Autodesk Inventor part; units mm, degrees
(part 3 of 3)
  line L418 (-54.6413, 55.359) -> (-49.6413, 64.0192) projected
  line L419 (-64.6413, 55.359) -> (-54.6413, 55.359) projected
  line L420 (-69.6413, 64.0192) -> (-64.6413, 55.359) projected
  line L421 (-64.6413, 72.6795) -> (-69.6413, 64.0192) projected
  line L422 (-25.981, 77.6795) -> (-15.981, 77.6795) projected
  line L423 (-30.981, 86.3397) -> (-25.981, 77.6795) projected
  line L424 (-25.981, 95) -> (-30.981, 86.3397) projected
  line L425 (-15.981, 95) -> (-25.981, 95) projected
  line L426 (-10.981, 86.3397) -> (-15.981, 95) projected
  line L427 (-15.981, 77.6795) -> (-10.981, 86.3397) projected
  line L428 (66.3397, 64.0192) -> (61.3397, 72.6795) projected
  line L429 (61.3397, 55.359) -> (66.3397, 64.0192) projected
  line L430 (51.3397, 55.359) -> (61.3397, 55.359) projected
  line L431 (46.3397, 64.0192) -> (51.3397, 55.359) projected
  line L432 (51.3397, 72.6795) -> (46.3397, 64.0192) projected
  line L433 (61.3397, 72.6795) -> (51.3397, 72.6795) projected
  line L434 (90, 77.6795) -> (100, 77.6795) projected
  line L435 (85, 86.3397) -> (90, 77.6795) projected
  line L436 (90, 95) -> (85, 86.3397) projected
  line L437 (100, 95) -> (90, 95) projected
  line L438 (105, 86.3397) -> (100, 95) projected
  line L439 (100, 77.6795) -> (105, 86.3397) projected
  line L440 (22.6795, 33.0382) -> (27.6795, 41.6985) projected
  line L441 (12.6795, 33.0382) -> (22.6795, 33.0382) projected
  line L442 (7.6795, 41.6985) -> (12.6795, 33.0382) projected
  line L443 (12.6795, 50.3587) -> (7.6795, 41.6985) projected
  line L444 (22.6795, 50.3587) -> (12.6795, 50.3587) projected
  line L445 (27.6795, 41.6985) -> (22.6795, 50.3587) projected
  line L446 (61.3399, 33.0382) -> (66.3399, 41.6985) projected
  line L447 (51.3399, 33.0382) -> (61.3399, 33.0382) projected
  line L448 (46.3399, 41.6985) -> (51.3399, 33.0382) projected
  line L449 (51.3399, 50.3587) -> (46.3399, 41.6985) projected
  line L450 (61.3399, 50.3587) -> (51.3399, 50.3587) projected
  line L451 (66.3399, 41.6985) -> (61.3399, 50.3587) projected
  line L452 (-11.6509, 75.1795) -> (-6.6509, 66.5192) projected
  line L453 (-6.6509, 83.8397) -> (-11.6509, 75.1795) projected
  line L454 (3.3491, 83.8397) -> (-6.6509, 83.8397) projected
  line L455 (8.3491, 75.1795) -> (3.3491, 83.8397) projected
  line L456 (3.3491, 66.5192) -> (8.3491, 75.1795) projected
  line L457 (-6.6509, 66.5192) -> (3.3491, 66.5192) projected
  line L458 (-45.3111, 83.8397) -> (-50.3111, 75.1795) projected
  line L459 (-35.3111, 83.8397) -> (-45.3111, 83.8397) projected
  line L460 (-30.3111, 75.1795) -> (-35.3111, 83.8397) projected
  line L461 (-35.3111, 66.5192) -> (-30.3111, 75.1795) projected
  line L462 (-45.3111, 66.5192) -> (-35.3111, 66.5192) projected
  line L463 (-50.3111, 75.1795) -> (-45.3111, 66.5192) projected
  line L464 (42.0096, 66.5192) -> (47.0096, 75.1795) projected
  line L465 (32.0096, 66.5192) -> (42.0096, 66.5192) projected
  line L466 (27.0096, 75.1795) -> (32.0096, 66.5192) projected
  line L467 (32.0096, 83.8397) -> (27.0096, 75.1795) projected
  line L468 (42.0096, 83.8397) -> (32.0096, 83.8397) projected
  line L469 (47.0096, 75.1795) -> (42.0096, 83.8397) projected
  line L470 (80.6699, 66.5192) -> (85.6699, 75.1795) projected
  line L471 (70.6699, 66.5192) -> (80.6699, 66.5192) projected
  line L472 (65.6699, 75.1795) -> (70.6699, 66.5192) projected
  line L473 (70.6699, 83.8397) -> (65.6699, 75.1795) projected
  line L474 (80.6699, 83.8397) -> (70.6699, 83.8397) projected
  line L475 (85.6699, 75.1795) -> (80.6699, 83.8397) projected
  line L476 (22.6795, 72.6795) -> (12.6795, 72.6795) projected
  line L477 (27.6795, 64.0192) -> (22.6795, 72.6795) projected
  line L478 (22.6795, 55.359) -> (27.6795, 64.0192) projected
  line L479 (12.6795, 55.359) -> (22.6795, 55.359) projected
  line L480 (7.6795, 64.0192) -> (12.6795, 55.359) projected
  line L481 (12.6795, 72.6795) -> (7.6795, 64.0192) projected
  line L482 (-22.75, -78.5665) -> (-17.25, -78.5665) projected
  line L483 (-22.75, -78.566) -> (-22.75, -78.5665) projected
  line L484 (-25.981, -78.566) -> (-22.75, -78.566) projected
  line L485 (-30.981, -69.9058) -> (-25.981, -78.566) projected
  line L486 (-25.981, -61.2455) -> (-30.981, -69.9058) projected
  line L487 (-15.981, -61.2455) -> (-25.981, -61.2455) projected
  line L488 (-10.981, -69.9058) -> (-15.981, -61.2455) projected
  line L489 (-15.981, -78.566) -> (-10.981, -69.9058) projected
  line L490 (-17.25, -78.566) -> (-15.981, -78.566) projected
  line L491 (-64.6413, -78.566) -> (-54.6413, -78.566) projected
  line L492 (-69.6413, -69.9058) -> (-64.6413, -78.566) projected
  line L493 (-64.6413, -61.2455) -> (-69.6413, -69.9058) projected
  line L494 (-54.6413, -61.2455) -> (-64.6413, -61.2455) projected
  line L495 (-49.6413, -69.9058) -> (-54.6413, -61.2455) projected
  line L496 (-54.6413, -78.566) -> (-49.6413, -69.9058) projected
  line L497 (-103.3015, -78.566) -> (-93.3015, -78.566) projected
  line L498 (-108.3015, -69.9058) -> (-103.3015, -78.566) projected
  line L499 (-103.3015, -61.2455) -> (-108.3015, -69.9058) projected
  line L500 (-93.3015, -61.2455) -> (-103.3015, -61.2455) projected
  line L501 (-88.3015, -69.9058) -> (-93.3015, -61.2455) projected
  line L502 (-93.3015, -78.566) -> (-88.3015, -69.9058) projected
  line L503 (-93.3015, -83.5665) -> (-103.3015, -83.5665) projected
  line L504 (-88.3015, -92.2268) -> (-93.3015, -83.5665) projected
  line L505 (-92.7894, -100) -> (-88.3015, -92.2268) projected
  line L506 (-65.1534, -100) -> (-92.7894, -100) projected
  line L507 (-83.9714, -94.7273) -> (-87.0156, -100) projected
  line L508 (-73.9714, -94.7273) -> (-83.9714, -94.7273) projected
  line L509 (-70.9272, -100) -> (-73.9714, -94.7273) projected
  line L510 (-65.1534, -100) -> (-92.7894, -100) projected
  line L511 (-69.6413, -92.2268) -> (-65.1534, -100) projected
  line L512 (-64.6413, -83.5665) -> (-69.6413, -92.2268) projected
  line L513 (-54.6413, -83.5665) -> (-64.6413, -83.5665) projected
  line L514 (-49.6413, -92.2268) -> (-54.6413, -83.5665) projected
  line L515 (-54.1291, -100) -> (-49.6413, -92.2268) projected
  line L516 (-65.1534, -100) -> (-54.1291, -100) projected
  line L517 (-45.3111, -94.7273) -> (-48.3553, -100) projected
  line L518 (-35.3111, -94.7273) -> (-45.3111, -94.7273) projected
  line L519 (-32.2669, -100) -> (-35.3111, -94.7273) projected
  line L520 (-26.4931, -100) -> (-92.7894, -100) projected
  line L521 (-30.981, -92.2268) -> (-26.4931, -100) projected
  line L522 (-25.981, -83.5665) -> (-30.981, -92.2268) projected
  line L523 (-15.981, -83.5665) -> (-25.981, -83.5665) projected
  line L524 (-10.981, -92.2268) -> (-15.981, -83.5665) projected
  line L525 (-15.4689, -100) -> (-10.981, -92.2268) projected
  line L526 (-65.1534, -100) -> (-15.4689, -100) projected
  line L527 (-6.6509, -94.7273) -> (-9.6951, -100) projected
  line L528 (3.3491, -94.7273) -> (-6.6509, -94.7273) projected
  line L529 (6.3933, -100) -> (3.3491, -94.7273) projected
  line L530 (12.1674, -100) -> (-92.7894, -100) projected
  line L531 (7.6795, -92.2268) -> (12.1674, -100) projected
  line L532 (12.6795, -83.5665) -> (7.6795, -92.2268) projected
  line L533 (22.6795, -83.5665) -> (12.6795, -83.5665) projected
  line L534 (27.6795, -92.2268) -> (22.6795, -83.5665) projected
  line L535 (23.1916, -100) -> (27.6795, -92.2268) projected
  line L536 (-65.1534, -100) -> (23.1916, -100) projected
  line L537 (32.0096, -94.7273) -> (28.9654, -100) projected
  line L538 (42.0096, -94.7273) -> (32.0096, -94.7273) projected
  line L539 (45.0538, -100) -> (42.0096, -94.7273) projected
  line L540 (50.8276, -100) -> (-92.7894, -100) projected
  line L541 (46.3397, -92.2268) -> (50.8276, -100) projected
  line L542 (51.3397, -83.5665) -> (46.3397, -92.2268) projected
  line L543 (61.3397, -83.5665) -> (51.3397, -83.5665) projected
  line L544 (66.3397, -92.2268) -> (61.3397, -83.5665) projected
  line L545 (61.8519, -100) -> (66.3397, -92.2268) projected
  line L546 (-65.1534, -100) -> (61.8519, -100) projected
  line L547 (70.6699, -94.7273) -> (67.6257, -100) projected
  line L548 (80.6699, -94.7273) -> (70.6699, -94.7273) projected
  line L549 (83.7141, -100) -> (80.6699, -94.7273) projected
  line L550 (89.4879, -100) -> (-92.7894, -100) projected
  line L551 (85, -92.2268) -> (89.4879, -100) projected
  line L552 (90, -83.5665) -> (85, -92.2268) projected
  line L553 (100, -83.5665) -> (90, -83.5665) projected
  line L554 (105, -92.2268) -> (100, -83.5665) projected
  line L555 (100.5121, -100) -> (105, -92.2268) projected
  line L556 (-65.1534, -100) -> (100.5121, -100) projected
  line L557 (109.3301, -94.7273) -> (106.2859, -100) projected
  line L558 (110, -94.7273) -> (109.3301, -94.7273) projected
  line L559 (110, 100) -> (110, -100) projected
  line L560 (109.3301, -89.7268) -> (110, -89.7268) projected
  line L561 (104.3301, -81.0665) -> (109.3301, -89.7268) projected
  line L562 (109.3301, -72.4063) -> (104.3301, -81.0665) projected
  line L563 (110, -72.4063) -> (109.3301, -72.4063) projected
  line L564 (110, 100) -> (110, -100) projected
  line L565 (109.3301, -67.4058) -> (110, -67.4058) projected
  line L566 (104.3301, -58.7455) -> (109.3301, -67.4058) projected
  line L567 (109.3301, -50.0853) -> (104.3301, -58.7455) projected
  line L568 (110, -50.0853) -> (109.3301, -50.0853) projected
  line L569 (110, 100) -> (110, -100) projected
  line L570 (109.3301, -45.0848) -> (110, -45.0848) projected
  line L571 (104.3301, -36.4245) -> (109.3301, -45.0848) projected
  line L572 (109.3301, -27.7643) -> (104.3301, -36.4245) projected
  line L573 (110, -27.7643) -> (109.3301, -27.7643) projected
  line L574 (110, 100) -> (110, -100) projected
  line L575 (109.3301, -22.7638) -> (110, -22.7638) projected
  line L576 (104.3301, -14.1035) -> (109.3301, -22.7638) projected
  line L577 (109.3301, -5.4433) -> (104.3301, -14.1035) projected
  line L578 (110, -5.4433) -> (109.3301, -5.4433) projected
  line L579 (110, 100) -> (110, -100) projected
  line L580 (109.3301, -0.4428) -> (110, -0.4428) projected
  line L581 (104.3301, 8.2175) -> (109.3301, -0.4428) projected
  line L582 (109.3301, 16.8777) -> (104.3301, 8.2175) projected
  line L583 (110, 16.8777) -> (109.3301, 16.8777) projected
  line L584 (110, 100) -> (110, -100) projected
  line L585 (109.3301, 21.8777) -> (110, 21.8777) projected
  line L586 (104.3301, 30.538) -> (109.3301, 21.8777) projected
  line L587 (109.3301, 39.1983) -> (104.3301, 30.538) projected
  line L588 (110, 39.1983) -> (109.3301, 39.1983) projected
  line L589 (110, 100) -> (110, -100) projected
  line L590 (109.3301, 44.1987) -> (110, 44.1987) projected
  line L591 (104.3301, 52.859) -> (109.3301, 44.1987) projected
  line L592 (109.3301, 61.5192) -> (104.3301, 52.859) projected
  line L593 (110, 61.5192) -> (109.3301, 61.5192) projected
  line L594 (110, 100) -> (110, -100) projected
  line L595 (109.3301, 66.5192) -> (110, 66.5192) projected
  line L596 (104.3301, 75.1795) -> (109.3301, 66.5192) projected
  line L597 (109.3301, 83.8397) -> (104.3301, 75.1795) projected
  line L598 (110, 83.8397) -> (109.3301, 83.8397) projected
  line L599 (110, 100) -> (110, -100) projected
  line L600 (109.3301, 88.8397) -> (110, 88.8397) projected
  line L601 (104.3301, 97.5) -> (109.3301, 88.8397) projected
  line L602 (105.7735, 100) -> (104.3301, 97.5) projected
  line L603 (84.2265, 100) -> (110, 100) projected
  line L604 (85.6699, 97.5) -> (84.2265, 100) projected
  line L605 (80.6699, 88.8397) -> (85.6699, 97.5) projected
  line L606 (70.6699, 88.8397) -> (80.6699, 88.8397) projected
  line L607 (65.6699, 97.5) -> (70.6699, 88.8397) projected
  line L608 (67.1132, 100) -> (65.6699, 97.5) projected
  line L609 (45.5662, 100) -> (67.1132, 100) projected
  line L610 (47.0096, 97.5) -> (45.5662, 100) projected
  line L611 (42.0096, 88.8397) -> (47.0096, 97.5) projected
  line L612 (32.0096, 88.8397) -> (42.0096, 88.8397) projected
  line L613 (27.0096, 97.5) -> (32.0096, 88.8397) projected
  line L614 (28.453, 100) -> (27.0096, 97.5) projected
  line L615 (6.9058, 100) -> (28.453, 100) projected
  line L616 (8.3491, 97.5) -> (6.9058, 100) projected
  line L617 (3.3491, 88.8397) -> (8.3491, 97.5) projected
  line L618 (-6.6509, 88.8397) -> (3.3491, 88.8397) projected
  line L619 (-11.6509, 97.5) -> (-6.6509, 88.8397) projected
  line L620 (-10.2075, 100) -> (-11.6509, 97.5) projected
  line L621 (-31.7545, 100) -> (-10.2075, 100) projected
  line L622 (-30.3111, 97.5) -> (-31.7545, 100) projected
  line L623 (-35.3111, 88.8397) -> (-30.3111, 97.5) projected
  line L624 (-45.3111, 88.8397) -> (-35.3111, 88.8397) projected
  line L625 (-50.3111, 97.5) -> (-45.3111, 88.8397) projected
  line L626 (-48.8678, 100) -> (-50.3111, 97.5) projected
  line L627 (-70, 100) -> (-48.8678, 100) projected
  line L628 (-70, 99.2816) -> (-70, 100) projected
  line L629 (-68.9714, 97.5) -> (-70, 99.2816) projected
  line L630 (-73.9714, 88.8397) -> (-68.9714, 97.5) projected
  line L631 (-83.9714, 88.8397) -> (-73.9714, 88.8397) projected
  line L632 (-88.9714, 97.5) -> (-83.9714, 88.8397) projected
  line L633 (-87.528, 100) -> (-88.9714, 97.5) projected
  line L634 (-93.3013, 100) -> (-87.528, 100) projected
  line L635 (-93.3014, 99.9998) -> (-93.3013, 100) projected
  line L636 (-103.3014, 99.9998) -> (-93.3014, 99.9998) projected
  line L637 (-103.3015, 100) -> (-103.3014, 99.9998) projected
  line L638 (-110, 100) -> (-103.3015, 100) projected
  line L639 (-110, 79.2821) -> (-110, 100) projected
  line L640 (-107.6314, 75.1795) -> (-110, 79.2821) projected
  line L641 (-110, 71.0769) -> (-107.6314, 75.1795) projected
  line L642 (-110, 12.3201) -> (-110, 71.0769) projected
  line L643 (-107.6314, 8.2175) -> (-110, 12.3201) projected
  line L644 (-110, 4.1149) -> (-107.6314, 8.2175) projected
  line L645 (-110, -10.0009) -> (-110, 4.1149) projected
  line L646 (-107.6314, -14.1035) -> (-110, -10.0009) projected
  line L647 (-110, -18.2061) -> (-107.6314, -14.1035) projected
  line L648 (-110, -32.3219) -> (-110, -18.2061) projected
  line L649 (-107.6314, -36.4245) -> (-110, -32.3219) projected
  line L650 (-110, -40.5271) -> (-107.6314, -36.4245) projected
  line L651 (-110, -54.6429) -> (-110, -40.5271) projected
  line L652 (-107.6314, -58.7455) -> (-110, -54.6429) projected
  line L653 (-110, -62.8481) -> (-107.6314, -58.7455) projected
  line L654 (-110, -76.9639) -> (-110, -62.8481) projected
  line L655 (-107.6314, -81.0665) -> (-110, -76.9639) projected
  line L656 (-110, -85.1691) -> (-107.6314, -81.0665) projected
  line L657 (-110, -99.2849) -> (-110, -85.1691) projected
  line L658 (-109.5872, -100) -> (-110, -99.2849) projected
  line L659 (-103.8136, -100) -> (-109.5872, -100) projected
  line L660 (-108.3015, -92.2268) -> (-103.8136, -100) projected
  line L661 (-103.3015, -83.5665) -> (-108.3015, -92.2268) projected
  line L662 (100, 72.6795) -> (90, 72.6795) projected
  line L663 (105, 64.0192) -> (100, 72.6795) projected
  line L664 (100, 55.359) -> (105, 64.0192) projected
  line L665 (90, 55.359) -> (100, 55.359) projected
  line L666 (85, 64.0192) -> (90, 55.359) projected
  line L667 (90, 72.6795) -> (85, 64.0192) projected
  line L668 (61.3397, 77.6795) -> (66.3397, 86.3397) projected
  line L669 (51.3397, 77.6795) -> (61.3397, 77.6795) projected
  line L670 (46.3397, 86.3397) -> (51.3397, 77.6795) projected
  line L671 (51.3397, 95) -> (46.3397, 86.3397) projected
  line L672 (61.3397, 95) -> (51.3397, 95) projected
  line L673 (66.3397, 86.3397) -> (61.3397, 95) projected
  line L674 (22.6795, 77.6795) -> (27.6795, 86.3397) projected
  line L675 (12.6795, 77.6795) -> (22.6795, 77.6795) projected
  line L676 (7.6795, 86.3397) -> (12.6795, 77.6795) projected
  line L677 (12.6795, 95) -> (7.6795, 86.3397) projected
  line L678 (22.6795, 95) -> (12.6795, 95) projected
  line L679 (27.6795, 86.3397) -> (22.6795, 95) projected
  line L680 (-15.981, 72.6795) -> (-25.981, 72.6795) projected
  line L681 (-10.981, 64.0192) -> (-15.981, 72.6795) projected
  line L682 (-15.981, 55.359) -> (-10.981, 64.0192) projected
  line L683 (-25.981, 55.359) -> (-15.981, 55.359) projected
  line L684 (-30.981, 64.0192) -> (-25.981, 55.359) projected
  line L685 (-25.981, 72.6795) -> (-30.981, 64.0192) projected
  line L686 (-64.6413, 77.6795) -> (-54.6413, 77.6795) projected
  line L687 (-69.6413, 86.3397) -> (-64.6413, 77.6795) projected
  line L688 (-64.6413, 95) -> (-69.6413, 86.3397) projected
  line L689 (-54.6413, 95) -> (-64.6413, 95) projected
  line L690 (-49.6413, 86.3397) -> (-54.6413, 95) projected
  line L691 (-54.6413, 77.6795) -> (-49.6413, 86.3397) projected
  line L692 (-93.3015, 72.6795) -> (-103.3015, 72.6795) projected
  line L693 (-88.3015, 64.0192) -> (-93.3015, 72.6795) projected
  line L694 (-93.3015, 55.359) -> (-88.3015, 64.0192) projected
  line L695 (-103.3015, 55.359) -> (-93.3015, 55.359) projected
  line L696 (-108.3015, 64.0192) -> (-103.3015, 55.359) projected
  line L697 (-103.3015, 72.6795) -> (-108.3015, 64.0192) projected
  line L698 (-73.9714, 39.1983) -> (-83.9714, 39.1983) projected
  line L699 (-70.4148, 33.038) -> (-73.9714, 39.1983) projected
  line L700 (-70, 33.038) -> (-70.4148, 33.038) projected
  line L701 (-70, 32.3196) -> (-70, 33.038) projected
  line L702 (-68.9714, 30.538) -> (-70, 32.3196) projected
  line L703 (-73.9714, 21.8777) -> (-68.9714, 30.538) projected
  line L704 (-83.9714, 21.8777) -> (-73.9714, 21.8777) projected
  line L705 (-88.9714, 30.538) -> (-83.9714, 21.8777) projected
  line L706 (-83.9714, 39.1983) -> (-88.9714, 30.538) projected
  line L707 (-35.3111, 39.1983) -> (-45.3111, 39.1983) projected
  line L708 (-30.3111, 30.538) -> (-35.3111, 39.1983) projected
  line L709 (-35.3111, 21.8777) -> (-30.3111, 30.538) projected
  line L710 (-45.3111, 21.8777) -> (-35.3111, 21.8777) projected
  line L711 (-50.3111, 30.538) -> (-45.3111, 21.8777) projected
  line L712 (-45.3111, 39.1983) -> (-50.3111, 30.538) projected
  line L713 (-6.6509, 44.1987) -> (3.3491, 44.1987) projected
  line L714 (-11.6509, 52.859) -> (-6.6509, 44.1987) projected
  line L715 (-6.6509, 61.5192) -> (-11.6509, 52.859) projected
  line L716 (3.3491, 61.5192) -> (-6.6509, 61.5192) projected
  line L717 (8.3491, 52.859) -> (3.3491, 61.5192) projected
  line L718 (3.3491, 44.1987) -> (8.3491, 52.859) projected
  line L719 (42.0096, 39.1983) -> (32.0096, 39.1983) projected
  line L720 (47.0096, 30.538) -> (42.0096, 39.1983) projected
  line L721 (42.0096, 21.8777) -> (47.0096, 30.538) projected
  line L722 (32.0096, 21.8777) -> (42.0096, 21.8777) projected
  line L723 (27.0096, 30.538) -> (32.0096, 21.8777) projected
  line L724 (32.0096, 39.1983) -> (27.0096, 30.538) projected
  line L725 (80.6699, 39.1983) -> (70.6699, 39.1983) projected
  line L726 (85.6699, 30.538) -> (80.6699, 39.1983) projected
  line L727 (80.6699, 21.8777) -> (85.6699, 30.538) projected
  line L728 (70.6699, 21.8777) -> (80.6699, 21.8777) projected
  line L729 (65.6699, 30.538) -> (70.6699, 21.8777) projected
  line L730 (70.6699, 39.1983) -> (65.6699, 30.538) projected
  point P0 (-70, -100)
  point P1 (-17.25, -84)
  point P2 (-17.25, -74)
  point P3 (-2.75, -39.5)
  point P4 (57.25, -79)
  point P5 (42.75, -34.5)
  point P6 (-17.25, -83.5665)
  dimension "d79" = 5
  dimension "d80" = 4.75
  dimension "d81" = 4.75
  dimension "d82" = 5
  dimension "d83" = 4.75
  dimension "d84" = 4.75
  dimension "d85" = 5
  constraints: 24 end point, 6 point on line, 5 parallel, 5 perpendicular, 4 horizontal, 3 vertical, 2 midpoint, 8 other
  measures "d79" distance between parallel lines of L2 L6
  measures "d80" distance between parallel lines of L10 L11
  measures "d81" distance from line of L12 point (-2.75, -39.5)
  measures "d82" distance between parallel lines of L12 L10
  measures "d83" distance from line of point (57.25, -79) L15
  measures "d84" distance between parallel lines of L17 L14
  measures "d85" distance between parallel lines of L15 L14
ref_plane "작업 평면1" through (0, 0, -5.5) normal (0, 0, -1) x (-1, 0, 0)
sketch "스케치5" plane through (0, 0, -5.5) normal (0, 0, -1) x (-1, 0, 0)
  line L0 (110, -95) -> (110, 95) projected
  line L1 (-70, 95) -> (-70, -95) projected
  line L2 (-7.5, -92.75) -> (-7.5, 92.75) projected
  line L3 (-70, -90.75) -> (110, -90.75)
  line L4 (110, -90.75) -> (110, -59.25)
  line L5 (110, -59.25) -> (-70, -59.25)
  line L6 (-70, -59.25) -> (-70, -90.75)
  line L7 (-70, -90.75) -> (110, -59.25) construction
  line L8 (110, -90.75) -> (-70, -59.25) construction
  arc A0 (16.25, -84) -> (23.75, -84) centre (20, -84) ccw projected
  arc A1 (23.75, -74) -> (16.25, -74) centre (20, -74) ccw projected
  circle A2 centre (-10, -69.25) radius 1.95
  circle A3 centre (-65, -64.25) radius 1.95
  circle A4 centre (-65, -95) radius 1.95
  circle A5 centre (-10, -90) radius 1.95
  line L9 (20, -111.2481) -> (20, -60.3206)
  circle A6 centre (50, -69.25) radius 1.95
  circle A7 centre (105, -64.25) radius 1.95
  circle A8 centre (105, -95) radius 1.95
  circle A9 centre (50, -90) radius 1.95
  line L10 (-65, -100) -> (105, -100) projected
  arc A10 (-63.75, -84) -> (-56.25, -84) centre (-60, -84) ccw projected
  arc A11 (-62.75, -84) -> (-57.25, -84) centre (-60, -84) ccw projected
  circle A12 centre (-10, -69.25) radius 3.5
  circle A13 centre (-10, -90) radius 3.5
  circle A14 centre (50, -69.25) radius 3.5
  circle A15 centre (50, -90) radius 3.5
  arc A16 (-70, -95) -> (-65, -100) centre (-65, -95) ccw projected
  line L11 (-14.75, -95) -> (-62.75, -95) projected
  circle A17 centre (-65, -64.25) radius 3.5
  circle A18 centre (-65, -95) radius 3.5
  circle A19 centre (105, -64.25) radius 3.5
  circle A20 centre (105, -95) radius 3.5
  point P0 (0, 0)
  point P1 (20, -75)
  point P2 (20, -87.75)
  point P3 (20, -70.25)
  point P4 (-60, -87.75)
  point P5 (-60, -86.75)
  dimension "d126" = 3
  dimension "d127" = 11
  dimension "d128" = 180
  dimension "d129" = 3.9
  dimension "d130" = 2.5
  dimension "d131" = 10
  dimension "d132" = 3.9
  dimension "d133" = 5
  dimension "d134" = 5
  dimension "d135" = 3.9
  dimension "d138" = 3.9
  dimension "d140" = 2.5
  dimension "d143" = 5
  dimension "d144" = 5
  dimension "d145" = 10
  dimension "d147" = 40.75
  dimension "d148" = 12.25
  dimension "d149" = 13.25
  dimension "d150" = 7
  dimension "d151" = 7
  dimension "d152" = 60
  dimension "d155" = 8.25
  dimension "d156" = 7
  dimension "d157" = 7
  constraints: 16 centre point, 14 end point, 8 symmetric about line, 4 coincident, 4 point on circle, 2 midpoint, 2 parallel, 1 horizontal, 1 perpendicular, 1 point on line, 1 vertical, 8 other
  measures "d126" distance from line of point (20, -87.75) L3
  measures "d127" distance from line of point (20, -70.25) L5
  measures "d128" distance of L4.end L5.end
  measures "d129" diameter of A2
  measures "d130" distance from line of L2 A2.centre
  measures "d131" distance from line of L5 A2.centre
  measures "d132" diameter of A3
  measures "d133" distance from line of L1 A3.centre
  measures "d134" distance from line of L5 A3.centre
  measures "d135" diameter of A4
  measures "d138" diameter of A5
  measures "d140" distance from line of L2 A5.centre
  measures "d143" distance of A4.centre L10.start
  measures "d144" distance from line of L1 A4.centre
  measures "d145" distance from line of L10 A5.centre
  measures "d147" distance between parallel lines of L10 L5
  measures "d148" distance from line of point (-60, -87.75) L10
  measures "d149" distance from line of L10 point (-60, -86.75)
  measures "d150" diameter of A12
  measures "d151" diameter of A13
  measures "d152" diameter of A2.centre L9
  measures "d155" distance from line of L11 point (-60, -86.75)
  measures "d156" diameter of A17
  measures "d157" diameter of A18
sketch "스케치6" plane through (0, 0, 5) normal (0, 0, 1) x (1, 0, 0)
  line L0 (93.3015, 95) -> (103.3015, 95) projected
  line L1 (15.981, 95) -> (25.981, 95) projected
  line L2 (-100, 95) -> (-90, 95) projected
  line L3 (103.8136, -100) -> (109.5872, -100) projected
  line L4 (110, -99.2849) -> (110, -85.1691) projected
  line L5 (110, -76.9639) -> (110, -62.8481) projected
  line L6 (110, -54.6429) -> (110, -40.5271) projected
  line L7 (110, -32.3219) -> (110, -18.2061) projected
  line L8 (110, -10.0009) -> (110, 4.1149) projected
  line L9 (110, 12.3201) -> (110, 71.0769) projected
  line L10 (110, 79.2821) -> (110, 100) projected
  line L11 (110, 100) -> (103.3015, 100) projected
  line L12 (93.3013, 100) -> (87.528, 100) projected
  line L13 (70, 100) -> (48.8678, 100) projected
  line L14 (31.7545, 100) -> (10.2075, 100) projected
  line L15 (-6.9058, 100) -> (-28.453, 100) projected
  line L16 (-45.5662, 100) -> (-67.1132, 100) projected
  line L17 (-84.2265, 100) -> (-110, 100) projected
  line L18 (-110, 100) -> (-110, -100) projected
  line L19 (-110, 100) -> (-110, -100) projected
  line L20 (-110, 100) -> (-110, -100) projected
  line L21 (-110, 100) -> (-110, -100) projected
  line L22 (-110, 100) -> (-110, -100) projected
  line L23 (-110, 100) -> (-110, -100) projected
  line L24 (-110, 100) -> (-110, -100) projected
  line L25 (-110, 100) -> (-110, -100) projected
  line L26 (-110, 100) -> (-110, -100) projected
  line L27 (-110, -100) -> (-100.5121, -100) projected
  line L28 (-89.4879, -100) -> (-61.8519, -100) projected
  line L29 (-89.4879, -100) -> (-61.8519, -100) projected
  line L30 (-50.8276, -100) -> (-23.1916, -100) projected
  line L31 (-50.8276, -100) -> (-23.1916, -100) projected
  line L32 (-12.1674, -100) -> (15.4689, -100) projected
  line L33 (-12.1674, -100) -> (15.4689, -100) projected
  line L34 (26.4931, -100) -> (54.1291, -100) projected
  line L35 (26.4931, -100) -> (54.1291, -100) projected
  line L36 (65.1534, -100) -> (92.7894, -100) projected
  line L37 (65.1534, -100) -> (92.7894, -100) projected
  line L38 (-61.3397, 95) -> (-51.3397, 95) projected
  line L39 (-22.6795, 95) -> (-12.6795, 95) projected
  line L40 (54.6413, 95) -> (64.6413, 95) projected
  line L41 (-110, -100) -> (110, -100)
  line L42 (110, -100) -> (110, 100)
  line L43 (110, 100) -> (-110, 100)
  line L44 (-110, 100) -> (-110, -100)
  line L45 (-105, -95) -> (105, -95)
  line L46 (105, -95) -> (105, 95)
  line L47 (105, 95) -> (-105, 95)
  line L48 (-105, 95) -> (-105, -95)
  point P0 (-105.7735, 100)
  point P1 (-110, 88.8397)
  point P2 (-110, 83.8397)
  point P3 (-110, 66.5192)
  point P4 (-110, 61.5192)
  point P5 (-110, 44.1987)
  point P6 (-110, 39.1983)
  point P7 (-110, 21.8777)
  point P8 (-110, 16.8777)
  point P9 (-110, -0.4428)
  point P10 (-110, -5.4433)
  point P11 (-110, -22.7638)
  point P12 (-110, -27.7643)
  point P13 (-110, -45.0848)
  point P14 (-110, -50.0853)
  point P15 (-110, -67.4058)
  point P16 (-110, -72.4063)
  point P17 (-110, -89.7268)
  point P18 (-110, -94.7273)
  point P19 (-106.2859, -100)
  point P20 (-83.7141, -100)
  point P21 (-67.6257, -100)
  point P22 (-45.0538, -100)
  point P23 (-28.9654, -100)
  point P24 (-6.3933, -100)
  point P25 (9.6951, -100)
  point P26 (32.2669, -100)
  point P27 (48.3553, -100)
  point P28 (70.9272, -100)
  point P29 (87.0156, -100)
  point P30 (0, 0)
  point P31 (-28.453, 100)
  point P32 (-105.7735, 100)
  point P33 (-110, 88.8397)
  point P34 (-110, 83.8397)
  point P35 (-110, 66.5192)
  point P36 (-110, 61.5192)
  point P37 (-110, 44.1987)
  point P38 (-110, 39.1983)
  point P39 (-110, 21.8777)
  point P40 (-110, 16.8777)
  point P41 (-110, -0.4428)
  point P42 (-110, -5.4433)
  point P43 (-110, -22.7638)
  point P44 (-110, -27.7643)
  point P45 (-110, -45.0848)
  point P46 (-110, -50.0853)
  point P47 (-110, -67.4058)
  point P48 (-110, -72.4063)
  point P49 (-110, -89.7268)
  point P50 (-110, -94.7273)
  point P51 (-106.2859, -100)
  dimension "d229" = 5
  constraints: 12 end point, 2 parallel, 2 vertical, 1 horizontal, 1 perpendicular, 9 other
extrude "돌출10" add sketch "스케치6" against normal blind 15
sketch "스케치7" plane through (0, 0, 5) normal (0, 0, 1) x (1, 0, 0)
  line L0 (110, 100) -> (-110, 100) projected
  line L1 (-110, 100) -> (-110, -100) projected
  line L2 (17.25, -78.5665) -> (17.25, -78.566) projected
  line L3 (22.75, -78.566) -> (22.75, -78.5665) projected
  line L4 (-22.6795, 72.6795) -> (-12.6795, 72.6795) projected
  line L5 (-100, 74) -> (-100, 84) construction
  line L6 (-97.25, 74) -> (-97.25, 84)
  line L7 (-102.75, 84) -> (-102.75, 74)
  arc A0 (-102.75, 74) -> (-97.25, 74) centre (-100, 74) ccw
  arc A1 (-97.25, 84) -> (-102.75, 84) centre (-100, 84) ccw
  line L8 (-151.9966, 0) -> (190.7207, 0)
  line L9 (0, 184.6414) -> (0, -145.8855)
  line L10 (-95.25, 84) -> (-95.25, 74)
  arc A2 (-104.75, 74) -> (-95.25, 74) centre (-100, 74) ccw
  line L11 (-104.75, 74) -> (-104.75, 84)
  arc A3 (-95.25, 84) -> (-104.75, 84) centre (-100, 84) ccw
  arc A4 (-62.75, 74) -> (-57.25, 74) centre (-60, 74) ccw
  arc A5 (-64.75, 74) -> (-55.25, 74) centre (-60, 74) ccw
  line L12 (-64.75, 74) -> (-64.75, 84)
  line L13 (-57.25, 74) -> (-57.25, 84)
  line L14 (-55.25, 84) -> (-55.25, 74)
  line L15 (-62.75, 84) -> (-62.75, 74)
  line L16 (-60, 74) -> (-60, 84) construction
  arc A6 (-57.25, 84) -> (-62.75, 84) centre (-60, 84) ccw
  arc A7 (-55.25, 84) -> (-64.75, 84) centre (-60, 84) ccw
  arc A8 (-22.75, 74) -> (-17.25, 74) centre (-20, 74) ccw
  arc A9 (-24.75, 74) -> (-15.25, 74) centre (-20, 74) ccw
  line L17 (-24.75, 74) -> (-24.75, 84)
  line L18 (-17.25, 74) -> (-17.25, 84)
  line L19 (-15.25, 84) -> (-15.25, 74)
  line L20 (-22.75, 84) -> (-22.75, 74)
  line L21 (-20, 74) -> (-20, 84) construction
  arc A10 (-17.25, 84) -> (-22.75, 84) centre (-20, 84) ccw
  arc A11 (-15.25, 84) -> (-24.75, 84) centre (-20, 84) ccw
  arc A12 (17.25, 74) -> (22.75, 74) centre (20, 74) ccw
  arc A13 (15.25, 74) -> (24.75, 74) centre (20, 74) ccw
  line L22 (15.25, 74) -> (15.25, 84)
  line L23 (22.75, 74) -> (22.75, 84)
  line L24 (24.75, 84) -> (24.75, 74)
  line L25 (17.25, 84) -> (17.25, 74)
  line L26 (20, 74) -> (20, 84) construction
  arc A14 (22.75, 84) -> (17.25, 84) centre (20, 84) ccw
  arc A15 (24.75, 84) -> (15.25, 84) centre (20, 84) ccw
  arc A16 (57.25, 74) -> (62.75, 74) centre (60, 74) ccw
  arc A17 (55.25, 74) -> (64.75, 74) centre (60, 74) ccw
  line L27 (55.25, 74) -> (55.25, 84)
  line L28 (62.75, 74) -> (62.75, 84)
  line L29 (64.75, 84) -> (64.75, 74)
  line L30 (57.25, 84) -> (57.25, 74)
  line L31 (60, 74) -> (60, 84) construction
  arc A18 (62.75, 84) -> (57.25, 84) centre (60, 84) ccw
  arc A19 (64.75, 84) -> (55.25, 84) centre (60, 84) ccw
  arc A20 (97.25, 74) -> (102.75, 74) centre (100, 74) ccw
  arc A21 (95.25, 74) -> (104.75, 74) centre (100, 74) ccw
  line L32 (95.25, 74) -> (95.25, 84)
  line L33 (102.75, 74) -> (102.75, 84)
  line L34 (104.75, 84) -> (104.75, 74)
  line L35 (97.25, 84) -> (97.25, 74)
  line L36 (100, 74) -> (100, 84) construction
  arc A22 (102.75, 84) -> (97.25, 84) centre (100, 84) ccw
  arc A23 (104.75, 84) -> (95.25, 84) centre (100, 84) ccw
  arc A24 (-22.75, -5) -> (-17.25, -5) centre (-20, -5) ccw
  arc A25 (-24.75, -5) -> (-15.25, -5) centre (-20, -5) ccw
  arc A26 (-15.25, 5) -> (-24.75, 5) centre (-20, 5) ccw
  line L37 (-100, -5) -> (-100, 5) construction
  line L38 (-97.25, -5) -> (-97.25, 5)
  line L39 (-102.75, 5) -> (-102.75, -5)
  arc A27 (-102.75, -5) -> (-97.25, -5) centre (-100, -5) ccw
  line L40 (-95.25, 5) -> (-95.25, -5)
  arc A28 (-104.75, -5) -> (-95.25, -5) centre (-100, -5) ccw
  line L41 (-104.75, -5) -> (-104.75, 5)
  arc A29 (-95.25, 5) -> (-104.75, 5) centre (-100, 5) ccw
  arc A30 (-97.25, 5) -> (-102.75, 5) centre (-100, 5) ccw
  line L42 (-22.75, 5) -> (-22.75, -5)
  line L43 (-20, -5) -> (-20, 5) construction
  arc A31 (-17.25, 5) -> (-22.75, 5) centre (-20, 5) ccw
  line L44 (-15.25, 5) -> (-15.25, -5)
  line L45 (-17.25, -5) -> (-17.25, 5)
  line L46 (-24.75, -5) -> (-24.75, 5)
  line L47 (-64.75, -5) -> (-64.75, 5)
  line L48 (-62.75, 5) -> (-62.75, -5)
  line L49 (-60, -5) -> (-60, 5) construction
  arc A32 (-57.25, 5) -> (-62.75, 5) centre (-60, 5) ccw
  arc A33 (-55.25, 5) -> (-64.75, 5) centre (-60, 5) ccw
  line L50 (-57.25, -5) -> (-57.25, 5)
  line L51 (-55.25, 5) -> (-55.25, -5)
  arc A34 (-62.75, -5) -> (-57.25, -5) centre (-60, -5) ccw
  arc A35 (-64.75, -5) -> (-55.25, -5) centre (-60, -5) ccw
  line L52 (95.25, -5) -> (95.25, 5)
  line L53 (97.25, 5) -> (97.25, -5)
  line L54 (100, -5) -> (100, 5) construction
  line L55 (102.75, -5) -> (102.75, 5)
  arc A36 (102.75, 5) -> (97.25, 5) centre (100, 5) ccw
  arc A37 (104.75, 5) -> (95.25, 5) centre (100, 5) ccw
  line L56 (104.75, 5) -> (104.75, -5)
  arc A38 (97.25, -5) -> (102.75, -5) centre (100, -5) ccw
  arc A39 (95.25, -5) -> (104.75, -5) centre (100, -5) ccw
  line L57 (64.75, 5) -> (64.75, -5)
  line L58 (62.75, -5) -> (62.75, 5)
  line L59 (60, -5) -> (60, 5) construction
  arc A40 (64.75, 5) -> (55.25, 5) centre (60, 5) ccw
  line L60 (57.25, 5) -> (57.25, -5)
  line L61 (55.25, -5) -> (55.25, 5)
  arc A41 (57.25, -5) -> (62.75, -5) centre (60, -5) ccw
  arc A42 (55.25, -5) -> (64.75, -5) centre (60, -5) ccw
  arc A43 (62.75, 5) -> (57.25, 5) centre (60, 5) ccw
  line L62 (24.75, 5) -> (24.75, -5)
  arc A44 (17.25, -5) -> (22.75, -5) centre (20, -5) ccw
  arc A45 (15.25, -5) -> (24.75, -5) centre (20, -5) ccw
  line L63 (22.75, -5) -> (22.75, 5)
  line L64 (20, -5) -> (20, 5) construction
  line L65 (17.25, 5) -> (17.25, -5)
  arc A46 (22.75, 5) -> (17.25, 5) centre (20, 5) ccw
  line L66 (15.25, -5) -> (15.25, 5)
  arc A47 (24.75, 5) -> (15.25, 5) centre (20, 5) ccw
  arc A48 (-22.75, -84) -> (-17.25, -84) centre (-20, -84) ccw
  arc A49 (-24.75, -84) -> (-15.25, -84) centre (-20, -84) ccw
  arc A50 (-15.25, -74) -> (-24.75, -74) centre (-20, -74) ccw
  line L67 (-100, -84) -> (-100, -74) construction
  line L68 (-97.25, -84) -> (-97.25, -74)
  line L69 (-102.75, -74) -> (-102.75, -84)
  arc A51 (-102.75, -84) -> (-97.25, -84) centre (-100, -84) ccw
  line L70 (-95.25, -74) -> (-95.25, -84)
  arc A52 (-104.75, -84) -> (-95.25, -84) centre (-100, -84) ccw
  line L71 (-104.75, -84) -> (-104.75, -74)
  arc A53 (-95.25, -74) -> (-104.75, -74) centre (-100, -74) ccw
  arc A54 (-97.25, -74) -> (-102.75, -74) centre (-100, -74) ccw
  line L72 (-22.75, -74) -> (-22.75, -84)
  line L73 (-20, -84) -> (-20, -74) construction
  arc A55 (-17.25, -74) -> (-22.75, -74) centre (-20, -74) ccw
  line L74 (-15.25, -74) -> (-15.25, -84)
  line L75 (-17.25, -84) -> (-17.25, -74)
  line L76 (-24.75, -84) -> (-24.75, -74)
  line L77 (-64.75, -84) -> (-64.75, -74)
  line L78 (-62.75, -74) -> (-62.75, -84)
  line L79 (-60, -84) -> (-60, -74) construction
  arc A56 (-57.25, -74) -> (-62.75, -74) centre (-60, -74) ccw
  arc A57 (-55.25, -74) -> (-64.75, -74) centre (-60, -74) ccw
  line L80 (-57.25, -84) -> (-57.25, -74)
  line L81 (-55.25, -74) -> (-55.25, -84)
  arc A58 (-62.75, -84) -> (-57.25, -84) centre (-60, -84) ccw
  arc A59 (-64.75, -84) -> (-55.25, -84) centre (-60, -84) ccw
  line L82 (95.25, -84) -> (95.25, -74)
  line L83 (97.25, -74) -> (97.25, -84)
  line L84 (100, -84) -> (100, -74) construction
  line L85 (102.75, -84) -> (102.75, -74)
  arc A60 (102.75, -74) -> (97.25, -74) centre (100, -74) ccw
  arc A61 (104.75, -74) -> (95.25, -74) centre (100, -74) ccw
  line L86 (104.75, -74) -> (104.75, -84)
  arc A62 (97.25, -84) -> (102.75, -84) centre (100, -84) ccw
  arc A63 (95.25, -84) -> (104.75, -84) centre (100, -84) ccw
  line L87 (64.75, -74) -> (64.75, -84)
  line L88 (62.75, -84) -> (62.75, -74)
  line L89 (60, -84) -> (60, -74) construction
  arc A64 (64.75, -74) -> (55.25, -74) centre (60, -74) ccw
  line L90 (57.25, -74) -> (57.25, -84)
  line L91 (55.25, -84) -> (55.25, -74)
  arc A65 (57.25, -84) -> (62.75, -84) centre (60, -84) ccw
  arc A66 (55.25, -84) -> (64.75, -84) centre (60, -84) ccw
  arc A67 (62.75, -74) -> (57.25, -74) centre (60, -74) ccw
  line L92 (24.75, -74) -> (24.75, -84)
  arc A68 (17.25, -84) -> (22.75, -84) centre (20, -84) ccw
  arc A69 (15.25, -84) -> (24.75, -84) centre (20, -84) ccw
  line L93 (22.75, -84) -> (22.75, -74)
  line L94 (20, -84) -> (20, -74) construction
  line L95 (17.25, -74) -> (17.25, -84)
  arc A70 (22.75, -74) -> (17.25, -74) centre (20, -74) ccw
  line L96 (15.25, -84) -> (15.25, -74)
  arc A71 (24.75, -74) -> (15.25, -74) centre (20, -74) ccw
  line L97 (-80, 34.5) -> (-80, 44.5) construction
  line L98 (-77.25, 34.5) -> (-77.25, 44.5)
  line L99 (-82.75, 44.5) -> (-82.75, 34.5)
  arc A72 (-82.75, 34.5) -> (-77.25, 34.5) centre (-80, 34.5) ccw
  arc A73 (-77.25, 44.5) -> (-82.75, 44.5) centre (-80, 44.5) ccw
  line L100 (-75.25, 44.5) -> (-75.25, 34.5)
  arc A74 (-84.75, 34.5) -> (-75.25, 34.5) centre (-80, 34.5) ccw
  line L101 (-84.75, 34.5) -> (-84.75, 44.5)
  arc A75 (-75.25, 44.5) -> (-84.75, 44.5) centre (-80, 44.5) ccw
  line L102 (-35.25, 44.5) -> (-35.25, 34.5)
  line L103 (-42.75, 44.5) -> (-42.75, 34.5)
  line L104 (-37.25, 34.5) -> (-37.25, 44.5)
  line L105 (-44.75, 34.5) -> (-44.75, 44.5)
  line L106 (-40, 34.5) -> (-40, 44.5) construction
  arc A76 (-44.75, 34.5) -> (-35.25, 34.5) centre (-40, 34.5) ccw
  arc A77 (-42.75, 34.5) -> (-37.25, 34.5) centre (-40, 34.5) ccw
  arc A78 (-37.25, 44.5) -> (-42.75, 44.5) centre (-40, 44.5) ccw
  arc A79 (-35.25, 44.5) -> (-44.75, 44.5) centre (-40, 44.5) ccw
  line L107 (4.75, 44.5) -> (4.75, 34.5)
  line L108 (-2.75, 44.5) -> (-2.75, 34.5)
  line L109 (2.75, 34.5) -> (2.75, 44.5)
  line L110 (-4.75, 34.5) -> (-4.75, 44.5)
  line L111 (0, 34.5) -> (0, 44.5) construction
  arc A80 (-4.75, 34.5) -> (4.75, 34.5) centre (0, 34.5) ccw
  arc A81 (-2.75, 34.5) -> (2.75, 34.5) centre (0, 34.5) ccw
  arc A82 (2.75, 44.5) -> (-2.75, 44.5) centre (0, 44.5) ccw
  arc A83 (4.75, 44.5) -> (-4.75, 44.5) centre (0, 44.5) ccw
  line L112 (44.75, 44.5) -> (44.75, 34.5)
  line L113 (37.25, 44.5) -> (37.25, 34.5)
  line L114 (42.75, 34.5) -> (42.75, 44.5)
  line L115 (35.25, 34.5) -> (35.25, 44.5)
  line L116 (40, 34.5) -> (40, 44.5) construction
  arc A84 (35.25, 34.5) -> (44.75, 34.5) centre (40, 34.5) ccw
  arc A85 (37.25, 34.5) -> (42.75, 34.5) centre (40, 34.5) ccw
  arc A86 (42.75, 44.5) -> (37.25, 44.5) centre (40, 44.5) ccw
  arc A87 (44.75, 44.5) -> (35.25, 44.5) centre (40, 44.5) ccw
  line L117 (84.75, 44.5) -> (84.75, 34.5)
  line L118 (77.25, 44.5) -> (77.25, 34.5)
  line L119 (82.75, 34.5) -> (82.75, 44.5)
  line L120 (75.25, 34.5) -> (75.25, 44.5)
  line L121 (80, 34.5) -> (80, 44.5) construction
  arc A88 (75.25, 34.5) -> (84.75, 34.5) centre (80, 34.5) ccw
  arc A89 (77.25, 34.5) -> (82.75, 34.5) centre (80, 34.5) ccw
  arc A90 (82.75, 44.5) -> (77.25, 44.5) centre (80, 44.5) ccw
  arc A91 (84.75, 44.5) -> (75.25, 44.5) centre (80, 44.5) ccw
  line L122 (-2.75, -34.5) -> (-2.75, -44.5)
  line L123 (2.75, -44.5) -> (2.75, -34.5)
  line L124 (0, -44.5) -> (0, -34.5) construction
  arc A92 (-2.75, -44.5) -> (2.75, -44.5) centre (0, -44.5) ccw
  arc A93 (-4.75, -44.5) -> (4.75, -44.5) centre (0, -44.5) ccw
  line L125 (-4.75, -44.5) -> (-4.75, -34.5)
  arc A94 (2.75, -34.5) -> (-2.75, -34.5) centre (0, -34.5) ccw
  arc A95 (4.75, -34.5) -> (-4.75, -34.5) centre (0, -34.5) ccw
  arc A96 (37.25, -44.5) -> (42.75, -44.5) centre (40, -44.5) ccw
  arc A97 (35.25, -44.5) -> (44.75, -44.5) centre (40, -44.5) ccw
  line L126 (44.75, -34.5) -> (44.75, -44.5)
  line L127 (42.75, -44.5) -> (42.75, -34.5)
  line L128 (40, -44.5) -> (40, -34.5) construction
  line L129 (37.25, -34.5) -> (37.25, -44.5)
  arc A98 (42.75, -34.5) -> (37.25, -34.5) centre (40, -34.5) ccw
  arc A99 (44.75, -34.5) -> (35.25, -34.5) centre (40, -34.5) ccw
  line L130 (84.75, -34.5) -> (84.75, -44.5)
  line L131 (77.25, -34.5) -> (77.25, -44.5)
  line L132 (82.75, -44.5) -> (82.75, -34.5)
  line L133 (80, -44.5) -> (80, -34.5) construction
  line L134 (75.25, -44.5) -> (75.25, -34.5)
  arc A100 (77.25, -44.5) -> (82.75, -44.5) centre (80, -44.5) ccw
  arc A101 (75.25, -44.5) -> (84.75, -44.5) centre (80, -44.5) ccw
  arc A102 (82.75, -34.5) -> (77.25, -34.5) centre (80, -34.5) ccw
  arc A103 (84.75, -34.5) -> (75.25, -34.5) centre (80, -34.5) ccw
  line L135 (4.75, -34.5) -> (4.75, -44.5)
  line L136 (35.25, -44.5) -> (35.25, -34.5)
  line L137 (-35.25, -34.5) -> (-35.25, -44.5)
  line L138 (-44.75, -44.5) -> (-44.75, -34.5)
  line L139 (-42.75, -34.5) -> (-42.75, -44.5)
  line L140 (-37.25, -44.5) -> (-37.25, -34.5)
  line L141 (-40, -44.5) -> (-40, -34.5) construction
  arc A104 (-42.75, -44.5) -> (-37.25, -44.5) centre (-40, -44.5) ccw
  arc A105 (-44.75, -44.5) -> (-35.25, -44.5) centre (-40, -44.5) ccw
  arc A106 (-77.25, -34.5) -> (-82.75, -34.5) centre (-80, -34.5) ccw
  arc A107 (-75.25, -34.5) -> (-84.75, -34.5) centre (-80, -34.5) ccw
  line L142 (-75.25, -34.5) -> (-75.25, -44.5)
  line L143 (-77.25, -44.5) -> (-77.25, -34.5)
  line L144 (-80, -44.5) -> (-80, -34.5) construction
  line L145 (-82.75, -34.5) -> (-82.75, -44.5)
  line L146 (-84.75, -44.5) -> (-84.75, -34.5)
  arc A108 (-82.75, -44.5) -> (-77.25, -44.5) centre (-80, -44.5) ccw
  arc A109 (-84.75, -44.5) -> (-75.25, -44.5) centre (-80, -44.5) ccw
  arc A110 (-35.25, -34.5) -> (-44.75, -34.5) centre (-40, -34.5) ccw
  arc A111 (-37.25, -34.5) -> (-42.75, -34.5) centre (-40, -34.5) ccw
  line L147 (-105, -2.9428) -> (-100, 5.7175) projected
  line L148 (-104.75, -2.5097) -> (-105, -2.9428)
  line L149 (-100, -11.603) -> (-105, -2.9428) projected
  line L150 (-105, -2.9428) -> (-104.75, -3.3758)
  point P0 (0, 0)
  point P1 (-100, 79)
  point P2 (-100, 86.75)
  point P3 (-100, 71.25)
  point P4 (-60, 71.25)
  point P5 (-60, 79)
  point P6 (-60, 86.75)
  point P7 (-20, 71.25)
  point P8 (-20, 79)
  point P9 (-20, 86.75)
  point P10 (20, 71.25)
  point P11 (20, 79)
  point P12 (20, 86.75)
  point P13 (60, 71.25)
  point P14 (60, 79)
  point P15 (60, 86.75)
  point P16 (100, 71.25)
  point P17 (100, 79)
  point P18 (100, 86.75)
  point P19 (-20, -7.75)
  point P20 (-100, 0)
  point P21 (-100, -7.75)
  point P22 (-100, 7.75)
  point P23 (-20, 7.75)
  point P24 (-20, 0)
  point P25 (-60, 0)
  point P26 (-60, 7.75)
  point P27 (-60, -7.75)
  point P28 (100, 0)
  point P29 (100, -7.75)
  point P30 (100, 7.75)
  point P31 (60, 7.75)
  point P32 (60, 0)
  point P33 (60, -7.75)
  point P34 (20, -7.75)
  point P35 (20, 0)
  point P36 (20, 7.75)
  point P37 (-20, -86.75)
  point P38 (-100, -79)
  point P39 (-100, -86.75)
  point P40 (-100, -71.25)
  point P41 (-20, -71.25)
  point P42 (-20, -79)
  point P43 (-60, -79)
  point P44 (-60, -71.25)
  point P45 (-60, -86.75)
  point P46 (100, -79)
  point P47 (100, -86.75)
  point P48 (100, -71.25)
  point P49 (60, -71.25)
  point P50 (60, -79)
  point P51 (60, -86.75)
  point P52 (20, -86.75)
  point P53 (20, -79)
  point P54 (20, -71.25)
  point P55 (-80, 39.5)
  point P56 (-80, 47.25)
  point P57 (-80, 31.75)
  point P58 (-40, 39.5)
  point P59 (-40, 31.75)
  point P60 (-40, 47.25)
  point P61 (0, 39.5)
  point P62 (0, 31.75)
  point P63 (0, 47.25)
  point P64 (40, 39.5)
  point P65 (40, 31.75)
  point P66 (40, 47.25)
  point P67 (80, 39.5)
  point P68 (80, 31.75)
  point P69 (80, 47.25)
  point P70 (0, -39.5)
  point P71 (0, -47.25)
  point P72 (0, -31.75)
  point P73 (80, -31.75)
  point P74 (40, -47.25)
  point P75 (40, -39.5)
  point P76 (40, -31.75)
  point P77 (80, -39.5)
  point P78 (80, -47.25)
  point P79 (-40, -39.5)
  point P80 (-40, -47.25)
  point P81 (-80, -31.75)
  point P82 (-80, -39.5)
  point P83 (-80, -47.25)
  point P84 (-40, -31.75)
  point P85 (-17.5878, 72.6795)
  point P86 (-22.4122, 72.6795)
  point P87 (-17.25, 0)
  point P88 (-22.75, 0)
  dimension "d232" = 5.5
  dimension "d234" = 10
  dimension "d235" = 21
  dimension "d236" = 15.5
  dimension "d237" = 2
  dimension "d240" = 40
  dimension "d247" = 79
  dimension "d252" = 5.5
  dimension "d253" = 15.5
  dimension "d254" = 2
  dimension "d255" = 20
  dimension "d256" = 55
  dimension "d259" = 40
  dimension "d266" = 79
  constraints: 344 end point, 228 point on circle, 112 centre point, 8 tangent, 6 vertical, 4 horizontal, 4 parallel, 4 point on line, 2 midpoint, 1 collinear, 578 other
  measures "d232" distance between parallel lines of L7 L6
  measures "d234" distance between parallel lines of L1 L5
  measures "d235" distance from line of L0 point (-100, 79)
  measures "d236" distance of point (-100, 86.75) point (-100, 71.25)
  measures "d237" distance between parallel lines of L10 L6
  measures "d240" distance of point (-100, 71.25) point (-60, 71.25)
  measures "d247" distance of point (-20, 71.25) point (-20, -7.75)
  measures "d252" distance between parallel lines of L99 L98
  measures "d253" distance of point (-80, 47.25) point (-80, 31.75)
  measures "d254" distance between parallel lines of L100 L98
  measures "d255" distance from line of L5 point (-80, 39.5)
  measures "d256" vertical distance of point (-100, 86.75) point (-80, 31.75)
  measures "d259" distance of L99.start L103.start
  measures "d266" distance of L110.end L125.end
extrude "돌출11" add sketch "스케치7" against normal blind 5 contours A83 L107 A80 L9 A81 L109 A82 | L9 A82 L108 A81 A80 L110 A83 | L41 A29 L40 L8 L38 A30 L39 L147 | L8 L147 L41 | L147 L39 L8 | L8 L39 A27 L38 L40 A28 L149 L41 L147 | L41 L149 L147 | L149 A28 L41 | L44 A25 L46 L8 L42 A24 L45 | L8 L45 A31 L42 L46 A26 L44 | L47 A33 L51 L8 L50 A32 L48 | L8 L48 A34 L50 L51 A35 L47 | L4 A8 | L66 A47 L62 L8 L63 A46 L65 | L8 L65 A44 L63 L62 A45 L66 | L61 A40 L57 L8 L58 A43 L60 | L8 L60 A41 L58 L57 A42 L61 | L52 A37 L56 L8 L55 A36 L53 | L8 L53 A38 L55 L56 A39 L52 | A95 L135 A93 L9 A92 L123 A94 | L9 A94 L122 A92 A93 L125 A95 | L10 A2 L11 A3 | L12 A7 L14 A5 | L17 A11 L19 A9 | L22 A15 L24 A13 | L27 A19 L29 A17 | L32 A23 L34 A21 | L76 A50 L74 A49 | L70 A52 L71 A53 | L77 A57 L81 A59 | L82 A61 L86 A63 | L87 A66 L91 A64 | L92 A69 L96 A71 | L100 A74 L101 A75 | L102 A76 L105 A79 | L112 A84 L115 A87 | L117 A88 L120 A91 | L136 A99 L126 A97 | L130 A101 L134 A103 | L137 A105 L138 A110 | L142 A109 L146 A107
extrude "돌출12" cut sketch "스케치7" against normal blind 5 contours A82 L109 A81 L9 | L9 A81 L108 A82 | L39 A30 L38 L8 | L8 L38 A27 L39 | L45 A24 L42 L8 | L8 L42 A31 L45 | L48 A32 L50 L8 | L8 L50 A34 L48 | A8 L20 A10 L18 L4 | L4 A8 | A0 L7 A1 L6 | L65 A46 L63 L8 | L8 L63 A44 L65 | L60 A43 L58 L8 | L8 L58 A41 L60 | L53 A36 L55 L8 | L8 L55 A38 L53 | A94 L123 A92 L9 | L9 A92 L122 A94 | L15 A6 L13 A4 | L25 A14 L23 A12 | L30 A18 L28 A16 | L35 A22 L33 A20 | L72 A55 L75 A48 | A51 L69 A54 L68 | A56 L80 A58 L78 | A60 L85 A62 L83 | A65 L90 A67 L88 | L95 A70 L93 A68 | A72 L99 A73 L98 | A78 L104 A77 L103 | A86 L114 A85 L113 | A90 L119 A89 L118 | L129 A98 L127 A96 | A102 L132 A100 L131 | A111 L140 A104 L139 | L143 A108 L145 A106
equation "\"d20\" = d2"
equation "\"d81\" = d80"
equation "\"d83\" = d80"
equation "\"d84\" = d80"
equation "\"d21\" = d3"
